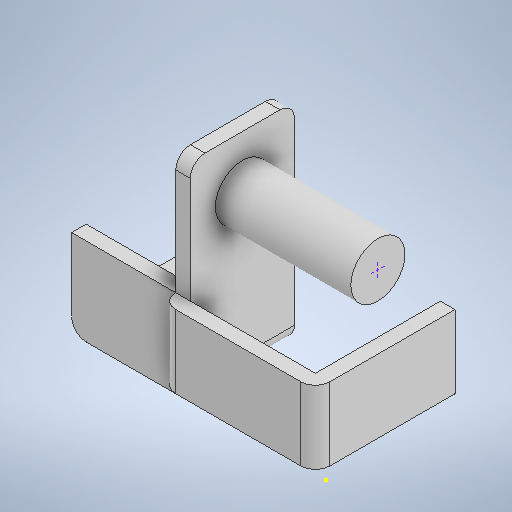
# Autodesk Inventor part: Sujetador2
Saved by Autodesk Inventor 2025.2 (Build 292293000, 293)
## iProperties
Created: 2025-05-13
Part Number: Sujetador2
Material: Generic
Document SubType Name: Modeling
Designer: USER
Density: 1 g/cm^3
Appearance: Default
Author: USER
Autodesk Inventor part; units mm, degrees
ref_plane "YZ Plane" through (0, 0, 0) normal (1, 0, 0) x (0, 1, 0)
ref_plane "XZ Plane" through (0, 0, 0) normal (0, 1, 0) x (-1, 0, 0)
ref_plane "XY Plane" through (0, 0, 0) normal (0, 0, 1) x (1, 0, 0)
sketch "Sketch1" plane through (0, 0, 0) normal (0, 1, 0) x (-1, 0, 0)
  line L0 (0, 0) -> (50, 0)
  line L1 (50, 0) -> (50, -50)
  line L2 (50, -50) -> (0, -50)
  line L3 (0, -50) -> (0, 0)
  dimension "d0" = 50
  dimension "d1" = 50
  constraints: 8 end point, 2 parallel, 1 horizontal, 1 perpendicular
  measures "d0" distance of L1.end L2.end
  measures "d1" distance of L0.end L1.end
extrude "Extrusion1" add sketch "Sketch1" along normal blind 7
sketch "Sketch2" plane through (0, 0, 0) normal (1, 0, 0) x (0, 0, -1)
  line L0 (0, 0) -> (50, 0)
  line L1 (50, 0) -> (50, 100)
  line L2 (50, 100) -> (0, 100)
  line L3 (0, 100) -> (0, 0)
  dimension "d4" = 100
  constraints: 8 end point, 2 parallel, 1 horizontal, 1 perpendicular
  measures "d4" distance of L1.end L0.end
extrude "Extrusion2" add sketch "Sketch2" along normal blind 7
sketch "Sketch3" plane through (7, 0, 0) normal (1, 0, 0) x (0, 0, -1)
  line L0 (50, 100) -> (0, 100) projected
  line L1 (25, 100) -> (25, 75)
  circle A0 centre (25, 75) radius 13
  point P0 (0, 0)
  dimension "d7" = 25
  dimension "d8" = 26
  constraints: 2 end point, 1 centre point, 1 coincident, 1 midpoint, 1 vertical
  measures "d7" distance of L1.start L1.end
  measures "d8" diameter of A0
extrude "Extrusion3" add sketch "Sketch3" along normal blind 65
sketch "Sketch4" plane through (-50, 0, 0) normal (0, 0, 1) x (1, 0, 0)
  line L0 (57, 100) -> (57, 0) projected
  line L1 (50, 7) -> (0, 7) projected
  line L2 (50, 7) -> (124, 7)
  line L3 (124, 7) -> (124, 42)
  line L4 (124, 42) -> (50, 42)
  line L5 (50, 42) -> (50, 7)
  dimension "d13" = 74
  dimension "d14" = 35
  constraints: 8 end point, 2 parallel, 1 horizontal, 1 perpendicular
  measures "d13" distance of L4.end L3.end
  measures "d14" distance of L3.end L2.end
extrude "Extrusion4" add sketch "Sketch4" along normal blind 7
sketch "Sketch5" plane through (-50, 0, 0) normal (0, 0, -1) x (-1, 0, 0)
  line L0 (-124, 7) -> (-124, 42) projected
  line L1 (-57, 7) -> (-124, 7) projected
  line L2 (-124, 42) -> (-117, 42)
  line L3 (-117, 42) -> (-117, 7)
  line L4 (-117, 7) -> (-124, 7)
  line L5 (-124, 7) -> (-124, 42)
  point P0 (-50, 0)
  dimension "d17" = 7
  constraints: 8 end point, 2 parallel, 1 horizontal, 1 perpendicular, 1 point on line
  measures "d17" distance of L3.end L4.end
extrude "Extrusion5" add sketch "Sketch5" along normal blind 60
fillet "Fillet1" radius 7 6 edges at (0, 24.5, 7) (-50, 0, -25) (74, 24.5, 7) (7, 0, -25) (3.5, 100, 0) (3.5, 100, -50)
sketch "Sketch6" plane through (72, 75, -25) normal (1, 0, 0) x (0, 0, -1)
  point P0 (-25, -75)
  point P1 (0, 0)
sketch "Sketch8" plane through (-43, 0, 0) normal (0, 0, 1) x (1, 0, 0)
  arc A0 (43, 0) -> (50, 7) centre (43, 7) ccw projected
  line L0 (50, 7) -> (43, 7) projected
  line L1 (-7, 7) -> (43, 7) projected
  arc A1 (-7, 7) -> (0, 0) centre (0, 7) ccw projected
  line L2 (0, 0) -> (43, 0) projected
  line L3 (43, 7) -> (-7, 7)
  line L4 (-7, 7) -> (-7, 42)
  line L5 (-7, 42) -> (43, 42)
  line L6 (43, 42) -> (43, 7)
  dimension "d24" = 35
  constraints: 8 end point, 2 parallel, 1 horizontal, 1 perpendicular
  measures "d24" distance of L3.end L4.end
extrude "Extrusion7" add sketch "Sketch8" against normal blind 7 contours L1 L4 L5 L6
body "Solid1"
